script OS top_v3 (Autodesk Fusion 360 design; units mm, degrees)
Autodesk Fusion 360 part; units mm, degrees
sketch "top content" plane through (0, 0, 0) normal (0, 0, 1) x (1, 0, 0)
  circle A0 centre (15, 105) radius 1.588
  circle A1 centre (15, 15) radius 1.588
  circle A2 centre (135, 105) radius 1.588
  line L0 (0, 120) -> (150, 120) construction
  line L1 (150, 120) -> (150, 0) construction
  line L2 (0, 120) -> (150, 0) construction
  line L3 (150, 0) -> (0, 0) construction
  circle A3 centre (130, 26.2849) radius 6.5
  circle A4 centre (20, 26.2849) radius 6.5
  circle A5 centre (75, 60) radius 1.588
  line L4 (150, 120) -> (0, 0) construction
  circle A6 centre (135, 15) radius 1.588
  circle A7 centre (75, 94.0002) radius 6.5
  line L5 (0, 0) -> (0, 120) construction
  line L6 (1.75, 0) -> (22.5, 0)
  line L7 (0, 1.75) -> (0, 22.5)
  circle A8 centre (30, 30) radius 1.588
  line L8 (10, 5) -> (140, 5)
  line L9 (145, 10) -> (145, 110)
  line L10 (140, 115) -> (10, 115)
  line L11 (5, 110) -> (5, 10)
  line L12 (5, 5) -> (145, 115) construction
  line L13 (145, 5) -> (5, 115) construction
  arc A9 (145, 110) -> (140, 115) centre (140, 110) ccw
  arc A10 (10, 115) -> (5, 110) centre (10, 110) ccw
  arc A11 (5, 10) -> (10, 5) centre (10, 10) ccw
  arc A12 (140, 5) -> (145, 10) centre (140, 10) ccw
  circle A13 centre (120, 30) radius 1.588
  circle A14 centre (30, 90) radius 1.588
  circle A15 centre (120, 90) radius 1.588
  point P0 (75, 60)
  point P1 (75, 60)
  point P2 (75, 60)
  dimension "d2090" = 120
  dimension "d2091" = 90
  dimension "d2092" = 150
  dimension "d2093" = 120
  dimension "d2094" = 13
  dimension "d2095" = 110
  dimension "d2096" = 3.176
  dimension "d2097" = 75
  dimension "d2101" = 20
  dimension "d2103" = 25.9998
  dimension "d2861" = 20
  dimension "d2862" = 26.2849
  dimension "d5914" = 15
  dimension "d5915" = 15
  dimension "d5916" = 3.176
  dimension "d5917" = 30
  dimension "d5918" = 30
  dimension "d5921" = 90
  dimension "d5922" = 60
  dimension "d5923" = 110
  dimension "d5924" = 140
  dimension "d5925" = 5
  dimension "d5926" = 5
  dimension "d5927" = 5
  dimension "d5928" = 5
  constraint perpendicular L0 L1
  constraint parallel L0 L3
  constraint parallel L1 L5
  constraint coincident P2 L2
  constraint coincident P2 L4
  constraint coincident P2 P1
  constraint equal A4 A7
  constraint equal A3 A4
  constraint horizontal L3
  constraint horizontal A4.centre A3.centre
  constraint collinear L3 L6
  constraint collinear L5 L7
  constraint horizontal L8
  constraint perpendicular L8 L9
  constraint parallel L8 L10
  constraint parallel L9 L11
  constraint coincident L12 P2
  constraint coincident L13 P2
  constraint coincident L12.end L10
  constraint coincident L12.end L9
  constraint tangent L10 A9
  constraint tangent L9 A9
  constraint coincident L13.end L11
  constraint coincident L13.end L10
  constraint tangent L11 A10
  constraint tangent L10 A10
  constraint coincident L12.start L11
  constraint coincident L12.start L8
  constraint tangent L11 A11
  constraint tangent L8 A11
  constraint coincident L13.start L8
  constraint coincident L13.start L9
  constraint tangent L8 A12
  constraint tangent L9 A12
  measures "d2092" distance of L0.start L0.end
  measures "d2093" distance of L0.start L3.end
  measures "d2094" diameter of A4
  measures "d2095" distance of A4.centre A3.centre
  measures "d2096" diameter of A1
  measures "d2097" distance of A7.centre L1
  measures "d2101" distance of A3.centre L1
  measures "d2103" distance of A7.centre L0
  measures "d2861" distance of A4.centre L5
  measures "d2862" distance of A4.centre L3
  measures "d5914" vertical distance of L3.end A1.centre
  measures "d5915" horizontal distance of L3.end A1.centre
  measures "d5916" diameter of A8
  measures "d5917" distance of L3 A8.centre
  measures "d5918" horizontal distance of L3.end A8.centre
  measures "d5923" distance of L13.start L12.end
  measures "d5924" distance of L12.end L13.end
  measures "d5925" radius of A9
  measures "d5926" radius of A10
  measures "d5927" radius of A11
  measures "d5928" radius of A12
sketch "b  stock" plane through (0, 0, 0) normal (0, 0, 1) x (1, 0, 0)
  line L0 (0, 0) -> (304.8, 0)
  line L1 (304.8, 0) -> (304.8, 609.6)
  line L2 (304.8, 609.6) -> (0, 609.6)
  line L3 (0, 609.6) -> (0, 0)
extrude "b  stock body extrude" add sketch "b  stock" along normal blind 3.175
equation "screwHoleSize = 3.176 mm"
equation "pcbMountHoles = 2 mm"
equation "d2090 = b_Length - 30 mm"
equation "d2091 = b_Depth - 30 mm"
equation "d2096 = screwHoleSize"
equation "b_Length = 150.00 mm" comment "Length (mm)"
equation "b_Depth = 120.00 mm" comment "Depth (mm)"
equation "b_Height = 65.00 mm" comment "Height (mm)"
equation "b_Thickness = 3.175 mm" comment "Thickness (mm)"
equation "b_Tool_diameter = 2.01 mm" comment "Tool Diameter (mm)"
equation "b_Tooth_width = 10.00 mm" comment "Target Tooth Width (mm)"
equation "b_Kerf = -0.16 mm" comment "Kerf (mm)- can be negative"
equation "b_Delta_from_bottom = -0.10 mm" comment "Additional fine adjustment of bone centers from bottom of holes(mm)- positive makes smaller bottom indents"
equation "b_Stock_x_dimension = 304.80 mm" comment "Stock X Dimension *"
equation "b_Stock_y_dimension = 609.60 mm" comment "Stock Y Dimension"
equation "b_Repeats_l_tmp = -1.00 mm" comment "temp hidden"
equation "Version_info = 0 mm" comment "1.2.0 LENGTH 150.0 DEPTH 120.0 HEIGHT 65.0 THICKNESS 3.175 TOOL_DIAMETER 2.01 TOOTH_WIDTH 10.0 KERF -0.16 DELTA_FROM_BOTTOM -0.1 STOCK_X_DIMENSION 304.8 STOCK_Y_DIMENSION 609.6 COMPONENT  REPEATS_L_TMP -1 CREATE_COMPONENTS False CREATE_BODIES 1 CREATE_EMPTY_CONTENTS False CREATE_CONSTRAINTS True CLEAR_PREVIOUSLY_GENERATED_ITEMS True JUST_CLEAR_PREVIOUSLY_GENERATED_ITEMS False CREATE_MANUFACTURING False JUST_CREATE_MANUFACTURING False DEBUG_JUST_ONE_PART False MANUAL_LAYOUT  LASER False JUST_BUILD_TEST False DEBUG True"
equation "d5916 = screwHoleSize"
equation "d5921 = b_Length - 60 mm"
equation "d5922 = b_Depth - 60 mm"
equation "d5923 = b_Depth - 10 mm"
equation "d5924 = b_Length - 10 mm"
named bodies: "b  stock body"
